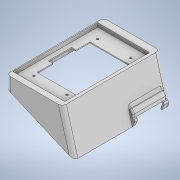
# Autodesk Inventor part: Front
Saved by Autodesk Inventor 2022 (Build 260153000, 153)
## iProperties
Created: 2021-06-27
Part Number: Front
Material: Generic
Document SubType Name: Modeling
Designer: Anton
Density: 1 g/cm^3
Appearance: Default
Author: Anton
Autodesk Inventor part; units mm, degrees
ref_plane "YZ Plane" through (0, 0, 0) normal (1, 0, 0) x (0, 1, 0)
ref_plane "XZ Plane" through (0, 0, 0) normal (0, 1, 0) x (-1, 0, 0)
ref_plane "XY Plane" through (0, 0, 0) normal (0, 0, 1) x (1, 0, 0)
sketch "Sketch1" plane through (0, 0, 0) normal (0, 1, 0) x (-1, 0, 0)
  line L0 (8, 0) -> (102.94, 0)
  line L1 (110.94, -8) -> (110.94, -185.2)
  line L2 (102.94, -193.2) -> (8, -193.2)
  line L3 (0, -185.2) -> (0, -8)
  circle A0 centre (88.297, -32) radius 2.1
  circle A1 centre (88.297, -158.2) radius 2.1
  circle A2 centre (22.6, -158.501) radius 2.1
  circle A3 centre (22.597, -32) radius 2.1
  arc A4 (110.94, -8) -> (102.94, 0) centre (102.94, -8) ccw
  arc A5 (8, 0) -> (0, -8) centre (8, -8) ccw
  arc A6 (0, -185.2) -> (8, -193.2) centre (8, -185.2) ccw
  arc A7 (102.94, -193.2) -> (110.94, -185.2) centre (102.94, -185.2) ccw
  point P0 (0, 0)
  dimension "d0" = 110.94
  dimension "d1" = 193.2
  dimension "d2" = 4.2
  dimension "d3" = 4.2
  dimension "d4" = 65.7
  dimension "d5" = 65.697
  dimension "d6" = 4.2
  dimension "d7" = 4.2
  dimension "d8" = 126.2
  dimension "d9" = 126.501
  dimension "d10" = 0
  dimension "d11" = 22.6
  dimension "d12" = 35
  dimension "d13" = 8
  dimension "d216" = 0
  dimension "d241" = 22.597
  constraints: 8 centre point, 8 end point, 8 point on circle, 8 tangent, 3 equal radius, 2 parallel, 2 point on line, 1 horizontal, 1 perpendicular
  measures "d0" distance between parallel lines of L3 L1
  measures "d1" distance between parallel lines of L2 L0
  measures "d2" diameter of A0
  measures "d3" diameter of A3
  measures "d4" distance of A3.centre A0.centre
  measures "d5" horizontal distance of A2.centre A1.centre
  measures "d6" diameter of A1
  measures "d7" diameter of A2
  measures "d8" distance of A1.centre A0.centre
  measures "d9" distance of A2.centre A3.centre
  measures "d10" vertical distance of A0.centre A3.centre
  measures "d11" distance from line of L3 A2.centre
  measures "d12" distance from line of L2 A1.centre
  measures "d13" radius of A4
  measures "d216" horizontal distance of A0.centre A1.centre
  measures "d241" distance from line of L3 A3.centre
extrude "Extrusion1" add sketch "Sketch1" along normal blind 2
sketch "Sketch2" plane through (0, 2, 0) normal (0, 1, 0) x (1, 0, 0)
  line L0 (-8, 193.2) -> (-102.94, 193.2) projected
  arc A0 (-102.94, 193.2) -> (-110.94, 185.2) centre (-102.94, 185.2) ccw projected
  line L1 (-110.94, 185.2) -> (-110.94, 8) projected
  arc A1 (-110.94, 8) -> (-102.94, 0) centre (-102.94, 8) ccw projected
  line L2 (-102.94, 0) -> (-8, 0) projected
  arc A2 (-8, 0) -> (0, 8) centre (-8, 8) ccw projected
  line L3 (0, 8) -> (0, 185.2) projected
  arc A3 (0, 185.2) -> (-8, 193.2) centre (-8, 185.2) ccw projected
  circle A4 centre (-88.297, 32) radius 2.1 projected
  circle A5 centre (-88.297, 158.2) radius 2.1 projected
  circle A6 centre (-22.6, 158.501) radius 2.1 projected
  circle A7 centre (-22.597, 32) radius 2.1 projected
  line L4 (-108.94, 11) -> (-108.94, 179.2)
  line L5 (-108.94, 179.2) -> (-6, 179.2)
  line L6 (-6, 11) -> (-108.94, 11)
  line L7 (-6, 179.2) -> (-6, 11)
  point P0 (0, 0)
  dimension "d16" = 2
  dimension "d17" = 14
  dimension "d18" = 11
  dimension "d19" = 6
  constraints: 8 end point, 1 horizontal
  measures "d16" distance between parallel lines of L1 L4
  measures "d17" distance between parallel lines of L0 L5
  measures "d18" distance between parallel lines of L2 L6
  measures "d19" distance between parallel lines of L3 L7
extrude "Extrusion2" add sketch "Sketch2" along normal blind 7.5 contours A3 L3 A2 L2 A1 L1 A0 L0
sketch "Sketch3" plane through (0, 2, 0) normal (0, 1, 0) x (1, 0, 0)
  line L0 (-91, 41) -> (-12, 41)
  line L1 (-12, 41) -> (-12, 146)
  line L2 (-12, 146) -> (-91, 146)
  line L3 (-6, 179.2) -> (-6, 11) projected
  line L4 (-6, 11) -> (-108.94, 11) projected
  line L5 (-99.94, 72) -> (-91, 72)
  line L6 (-91, 118.2) -> (-99.94, 118.2)
  line L7 (-99.94, 118.2) -> (-99.94, 72)
  circle A0 centre (-88.297, 158.2) radius 2.1 projected
  circle A1 centre (-88.297, 32) radius 2.1 projected
  line L8 (-108.94, 11) -> (-108.94, 179.2) projected
  line L9 (-91, 146) -> (-91, 118.2)
  line L10 (-91, 72) -> (-91, 41)
  point P0 (0, 0)
  dimension "d22" = 105
  dimension "d24" = 6
  dimension "d25" = 30
  dimension "d26" = 40
  dimension "d27" = 40
  dimension "d28" = 9
  constraints: 16 end point, 4 parallel, 2 horizontal, 1 perpendicular
  measures "d22" distance between parallel lines of L2 L0
  measures "d24" distance between parallel lines of L3 L1
  measures "d25" distance between parallel lines of L4 L0
  measures "d26" distance from line of L6 A0.centre
  measures "d27" distance from line of L5 A1.centre
  measures "d28" distance between parallel lines of L8 L7
extrude "Extrusion3" cut sketch "Sketch3" against normal blind 7.5 contours L10 L5 L7 L6 L9 L2 L1 L0
sketch "Sketch5" plane through (0, 0, 0) normal (0, -1, 0) x (1, 0, 0)
  line L0 (-12, -146) -> (-91, -146) projected
  line L1 (-91, -146) -> (-91, -118.2) projected
  line L2 (-91, -118.2) -> (-99.94, -118.2) projected
  line L3 (-99.94, -118.2) -> (-99.94, -72) projected
  line L4 (-99.94, -72) -> (-91, -72) projected
  line L5 (-91, -72) -> (-91, -41) projected
  line L6 (-91, -41) -> (-12, -41) projected
  line L7 (-12, -41) -> (-12, -146) projected
  line L8 (-8, -193.2) -> (-102.94, -193.2) projected
  arc A0 (-8, -193.2) -> (0, -185.2) centre (-8, -185.2) ccw projected
  line L9 (0, -8) -> (0, -185.2) projected
  arc A1 (0, -8) -> (-8, 0) centre (-8, -8) ccw projected
  line L10 (-102.94, 0) -> (-8, 0) projected
  arc A2 (-102.94, 0) -> (-110.94, -8) centre (-102.94, -8) ccw projected
  line L11 (-110.94, -185.2) -> (-110.94, -8) projected
  arc A3 (-110.94, -185.2) -> (-102.94, -193.2) centre (-102.94, -185.2) ccw projected
  circle A4 centre (-88.297, -32) radius 2.1 projected
  circle A5 centre (-88.297, -158.2) radius 2.1 projected
  circle A6 centre (-22.6, -158.501) radius 2.1 projected
  circle A7 centre (-22.597, -32) radius 2.1 projected
  line L12 (-102.94, -191.2) -> (-8, -191.2)
  arc A8 (-8, -191.2) -> (-2, -185.2) centre (-8, -185.2) ccw
  line L13 (-2, -185.2) -> (-2, -8)
  arc A9 (-2, -8) -> (-8, -2) centre (-8, -8) ccw
  line L14 (-8, -2) -> (-102.94, -2)
  arc A10 (-102.94, -2) -> (-108.94, -8) centre (-102.94, -8) ccw
  line L15 (-108.94, -8) -> (-108.94, -185.2)
  arc A11 (-108.94, -185.2) -> (-102.94, -191.2) centre (-102.94, -185.2) ccw
  point P0 (0, 0)
  dimension "d39" = 2
  constraints: 8 end point, 8 point on circle, 4 centre point, 7 other
  measures "d39" radial gap between concentric circles of A3 A11
extrude "Extrusion4" add sketch "Sketch5" along normal blind 72 contours L8 A3 L11 A2 L10 A1 L9 A0
sketch "Sketch6" plane through (-8, 9.5, -193.2) normal (0, 0, -1) x (-1, 0, 0)
  line L0 (102.94, -81.5) -> (102.94, 0)
  line L1 (-8, -81.5) -> (102.94, -81.5)
  line L2 (102.94, -81.5) -> (102.94, -23.5)
  line L3 (102.94, 0) -> (94.94, 0)
  line L4 (-8, -81.5) -> (0, -81.5)
  line L5 (0, 0) -> (-8, 0)
  line L6 (0, 0) -> (94.94, 0)
  line L7 (102.94, -23.5) -> (-25.549035, -79.092876)
  line L8 (-8, -81.5) -> (-29.89843, -81.5)
  line L9 (-29.89843, -81.5) -> (-31.1125, -81.5)
  line L10 (-25.549035, -79.092876) -> (-31.1125, -81.5)
  line L11 (-8, -81.5) -> (-8, 0)
  point P0 (-8, -9.5)
  dimension "d42" = 23.5
  dimension "d47" = 23.3965
  dimension "d48" = 140
  dimension "d51" = 23.1125
  constraints: 12 end point, 3 horizontal, 1 point on line
  measures "d42" distance from line of L3 L2.end
  measures "d47" angle of L6 L7
  measures "d48" distance of L2.end L7.end
  measures "d51" distance from line of L9.end L11
extrude "Extrusion5" cut sketch "Sketch6" along normal mid plane 1000 contours L1 L11 L7 L0 | L11 L8 L9 L10 L7
sketch "Sketch7" plane through (0, 9.5, 0) normal (0, 1, 0) x (1, 0, 0)
  arc A0 (-102.94, 193.2) -> (-110.94, 185.2) centre (-102.94, 185.2) ccw projected
  line L0 (-110.94, 185.2) -> (-110.94, 8) projected
  arc A1 (-110.94, 8) -> (-102.94, 0) centre (-102.94, 8) ccw projected
  line L1 (-102.94, 0) -> (-8, 0) projected
  arc A2 (-8, 0) -> (0, 8) centre (-8, 8) ccw projected
  line L2 (0, 8) -> (0, 185.2) projected
  arc A3 (0, 185.2) -> (-8, 193.2) centre (-8, 185.2) ccw projected
  line L3 (-8, 193.2) -> (-102.94, 193.2) projected
  line L4 (-108.94, 11) -> (-108.94, 179.2) projected
  line L5 (-108.94, 179.2) -> (-6, 179.2) projected
  line L6 (-6, 179.2) -> (-6, 11) projected
  line L7 (-6, 11) -> (-108.94, 11) projected
  line L8 (-8, 0) -> (23.113, 0)
  arc A4 (-8, 0) -> (0, 8) centre (-8, 8) ccw projected
  line L9 (23.113, 0) -> (23.113, 193.2)
  line L10 (23.113, 193.2) -> (-8, 193.2)
  arc A5 (0, 185.2) -> (-8, 193.2) centre (-8, 185.2) ccw projected
  point P0 (0, 0)
  point P1 (-8, 193.2)
  dimension "d52" = 23.113
  constraints: 6 end point, 2 perpendicular, 2 point on circle, 2 tangent, 1 horizontal
  measures "d52" distance between parallel lines of L2 L9
extrude "Extrusion6" add sketch "Sketch7" against normal up to surface contours L10 L9 L8 A2 L2 A3 surface through (-110.94, -14, -193.2) normal (0.397092, 0.9177788, 0)
sketch "Sketch8" plane through (-102.94, -17.46133, 0) normal (0, 0, 1) x (1, 0, 0)
  line L0 (126.053, 26.96133) -> (0, 26.96133)
  line L1 (126.053, 26.96133) -> (102.94, 26.96133)
  line L2 (0, 0) -> (126.053, -54.538886)
  line L3 (102.94, 26.96133) -> (126.053, -54.538886)
  line L4 (126.053, 26.96133) -> (126.053, -54.538886)
  line L5 (126.053, -54.538886) -> (126.053, 26.96133)
  point P0 (102.94, 17.46133)
  point P1 (96.94, 26.96133)
  dimension "d55" = 6
  constraints: 6 end point, 1 collinear, 1 point on line
  measures "d55" distance of point (96.94, 26.961) L1.end
extrude "Extrusion7" cut sketch "Sketch8" against normal blind 1000
sketch "Sketch9" plane through (0, 9.5, 0) normal (0, 1, 0) x (1, 0, 0)
  line L0 (23.113, 0) -> (0, 0) projected
  line L1 (-8, 0) -> (-110.94, 0)
  line L2 (-110.94, 0) -> (-110.94, 193.2)
  line L3 (-110.94, 193.2) -> (-8, 193.2)
  line L4 (0, 185.2) -> (0, 8)
  arc A0 (0, 185.2) -> (-8, 193.2) centre (-8, 185.2) ccw
  arc A1 (-8, 0) -> (0, 8) centre (-8, 8) ccw
  line L5 (0, 0) -> (0, 193.2) projected
  line L6 (0, 193.2) -> (0, 185.2)
  line L7 (-8, 193.2) -> (0, 193.2)
  line L8 (-102.94, 193.2) -> (23.113, 193.2) projected
  line L9 (-8, 0) -> (0, 0)
  line L10 (23.113, 0) -> (-102.94, 0) projected
  line L11 (0, 8) -> (0, 0)
  dimension "d58" = 8
  constraints: 16 end point, 6 tangent, 5 point on circle, 3 point on line, 2 centre point, 2 collinear, 2 parallel, 2 perpendicular, 1 equal radius, 1 horizontal
  measures "d58" radius of A0
sketch3d "3D Sketch1"
  line L0 (0, 9.5, 0) -> (23.113, -72.000216, 0)
sweep "Sweep1" cut profiles "Sketch9" path "3D Sketch1" contours A1 L5 L9 | A0 L7 L5
ref_plane "Work Plane1" through (23.113, -72.000216, -144.9) normal (-0.272835, 0.9620608, 0) x (0, 0, 1)
sketch "Sketch11" plane through (23.113, -72.000216, -144.9) normal (-0.272835, 0.9620608, 0) x (0, 0, 1)
  line L0 (-46.3, -106.390538) -> (-46.3, -26.259818)
  ellipse E0 centre (-40.3, -106.390538) end of major axis (-34.3, -106.390538) minor radius 5.064086 (-46.3, -106.390538) -> (-40.3, -111.454624) ccw
  line L1 (136.9, -111.454624) -> (-40.3, -111.454624)
  ellipse E1 centre (136.9, -106.390538) end of major axis (142.9, -106.390538) minor radius 5.064086 (136.9, -111.454624) -> (142.9, -106.390538) ccw
  line L2 (142.9, -26.259818) -> (142.9, -106.390538)
  ellipse E2 centre (136.9, -26.259818) end of major axis (130.9, -26.259818) minor radius 5.064086 (142.9, -26.259818) -> (136.9, -21.195732) ccw
  line L3 (-40.3, -21.195732) -> (136.9, -21.195732)
  ellipse E3 centre (-40.3, -26.259818) end of major axis (-46.3, -26.259818) minor radius 5.064086 (-40.3, -21.195732) -> (-46.3, -26.259818) ccw
  ellipse E4 centre (-40.3, -7.696487) end of major axis (-48.3, -7.696487) minor radius 7.696487 (-40.3, 0) -> (-48.3, -7.696487) ccw
  line L4 (-40.3, 0) -> (136.9, 0)
  ellipse E5 centre (136.9, -7.696487) end of major axis (144.9, -7.696487) minor radius 7.696487 (144.9, -7.696487) -> (136.9, 0) ccw
  line L5 (144.9, -7.696487) -> (144.9, -106.390538)
  ellipse E6 centre (136.9, -106.390538) end of major axis (144.9, -106.390538) minor radius 6.752115 (136.9, -113.142652) -> (144.9, -106.390538) ccw
  line L6 (-40.3, -113.142652) -> (136.9, -113.142652)
  ellipse E7 centre (-40.3, -106.390538) end of major axis (-32.3, -106.390538) minor radius 6.752115 (-48.3, -106.390538) -> (-40.3, -113.142652) ccw
  line L7 (-48.3, -106.390538) -> (-48.3, -7.696487)
  line L8 (142.9, -106.390538) -> (142.9, -7.696487)
  line L9 (136.9, -2) -> (-40.3, -2)
  line L10 (-46.3, -7.696487) -> (-46.3, -106.390538)
  line L11 (-40.3, -111.142652) -> (136.9, -111.142652)
  spline S0 degree 5 poles (142.900027, -7.696487) (142.900072, -6.800566) (142.71432, -5.904846) (142.342732, -5.060866) (141.262105, -3.534216) (139.68167, -2.526209) (138.783342, -2.175495) (137.841626, -2.000059) (136.9, -2.000018) knots 0 0 0 0 0 0 0.48753596 0.48753596 0.48753596 1 1 1 1 1 1
  spline S1 degree 5 poles (-40.3, -2.000018) (-41.241626, -2.000059) (-42.183342, -2.175495) (-43.08167, -2.526209) (-44.662105, -3.534216) (-45.742732, -5.060866) (-46.11432, -5.904846) (-46.300072, -6.800566) (-46.300027, -7.696487) knots 0 0 0 0 0 0 0.51246404 0.51246404 0.51246404 1 1 1 1 1 1
  spline S2 degree 5 poles (-46.300028, -106.390538) (-46.299997, -106.793405) (-46.245041, -107.196193) (-46.135378, -107.589075) (-45.689147, -108.646938) (-44.917064, -109.520861) (-44.327938, -109.984476) (-43.197488, -110.630825) (-41.951018, -110.989571) (-41.404874, -111.091631) (-40.852448, -111.14266) (-40.3, -111.142659) knots 0 0 0 0 0 0 0.23795953 0.23795953 0.23795953 0.67370232 0.67370232 0.67370232 1 1 1 1 1 1
  spline S3 degree 5 poles (136.9, -111.142659) (137.452448, -111.14266) (138.004874, -111.091631) (138.551018, -110.989571) (139.797488, -110.630825) (140.927938, -109.984476) (141.517064, -109.520861) (142.289147, -108.646938) (142.735378, -107.589075) (142.845041, -107.196193) (142.899997, -106.793405) (142.900028, -106.390538) knots 0 0 0 0 0 0 0.32629768 0.32629768 0.32629768 0.76204047 0.76204047 0.76204047 1 1 1 1 1 1
  point P0 (-46.3, -26.259818)
  dimension "d64" = 2
  constraints: 8 end point, 7 parallel, 20 other
  measures "d64" distance between parallel lines of L5 L8
extrude "Extrusion8" cut sketch "Sketch11" along normal up to surface contours L10 S1 L9 S0 L8 E2 L3 E3 surface through (-55.47, 0, -96.6) normal (0, 1, 0)
sketch "Sketch13" plane through (-110.94, -14, -185.2) normal (-0.397092, -0.9177788, 0) x (0.9177788, -0.397092, 0)
  line L0 (8.716697, -6) -> (136.126583, -6)
  ellipse E0 centre (8.716697, 0) end of major axis (15.25422, 0) minor radius 6 (2.179174, 0) -> (8.716697, -6) ccw
  line L1 (2.179174, 177.2) -> (2.179174, 0)
  ellipse E1 centre (8.716697, 177.2) end of major axis (15.25422, 177.2) minor radius 6 (8.716697, 183.2) -> (2.179174, 177.2) ccw
  line L2 (136.126583, 183.2) -> (8.716697, 183.2)
  spline S0 degree 7 poles (136.126583, 183.2) (136.514527, 183.200024) (136.902423, 183.180536) (137.289504, 183.141539) (137.674916, 183.082885) (138.05772, 183.004312) (138.436886, 182.905417) (139.157072, 182.674889) (139.498675, 182.546371) (139.835263, 182.39953) (140.165705, 182.233761) (140.488576, 182.048389) (140.802158, 181.842677) (141.299115, 181.469659) (141.489055, 181.314781) (141.673712, 181.15096) (141.852403, 180.977999) (142.024338, 180.795762) (142.188611, 180.604159) (142.457675, 180.256647) (142.566512, 180.105147) (142.670337, 179.948687) (142.768711, 179.787325) (142.861165, 179.621174) (142.947212, 179.450415) (143.149707, 179.002474) (143.25641, 178.71888) (143.344447, 178.425849) (143.412009, 178.125078) (143.457652, 177.818689) (143.480468, 177.509274) (143.480485, 177.2) knots 0 0 0 0 0 0 0 0 0.27563178 0.27563178 0.27563178 0.27563178 0.27563178 0.27563178 0.53020731 0.53020731 0.53020731 0.53020731 0.53020731 0.53020731 0.69417397 0.69417397 0.69417397 0.69417397 0.69417397 0.69417397 0.81372113 0.81372113 0.81372113 0.81372113 0.81372113 0.81372113 1 1 1 1 1 1 1 1
  line L3 (143.480508, 177.2) -> (143.480508, 0)
  spline S1 degree 7 poles (143.480508, 0) (143.480483, -0.309687) (143.457602, -0.619514) (143.411833, -0.926303) (143.344092, -1.227451) (143.255827, -1.520831) (143.148856, -1.804739) (142.945718, -2.253474) (142.859288, -2.424717) (142.766416, -2.591318) (142.667593, -2.753097) (142.563293, -2.90994) (142.453959, -3.06179) (142.184771, -3.408634) (142.020977, -3.599324) (141.849593, -3.780721) (141.671514, -3.952914) (141.487519, -4.116038) (141.298284, -4.270288) (140.803097, -4.641965) (140.49062, -4.847042) (140.168911, -5.031915) (139.839673, -5.197313) (139.504316, -5.343906) (139.163963, -5.472292) (138.443965, -5.703569) (138.063676, -5.80309) (137.679713, -5.882159) (137.293117, -5.941182) (136.904837, -5.980426) (136.515735, -6.000042) (136.126583, -6.000027) knots 0 0 0 0 0 0 0 0 0.18652709 0.18652709 0.18652709 0.18652709 0.18652709 0.18652709 0.30646281 0.30646281 0.30646281 0.30646281 0.30646281 0.30646281 0.46980351 0.46980351 0.46980351 0.46980351 0.46980351 0.46980351 0.72351021 0.72351021 0.72351021 0.72351021 0.72351021 0.72351021 1 1 1 1 1 1 1 1
  ellipse E2 centre (136.126583, 0) end of major axis (126.190741, 0) minor radius 8 (136.126583, -8) -> (146.062425, 0) ccw
  line L4 (146.062425, 0) -> (146.062425, 177.2)
  ellipse E3 centre (136.126583, 177.2) end of major axis (146.062425, 177.2) minor radius 8 (146.062425, 177.2) -> (136.126583, 185.2) ccw
  line L5 (136.126583, 185.2) -> (8.716697, 185.2)
  ellipse E4 centre (8.716697, 177.2) end of major axis (0, 177.2) minor radius 8 (8.716697, 185.2) -> (0, 177.2) ccw
  line L6 (0, 0) -> (0, 177.2)
  ellipse E5 centre (8.716697, 0) end of major axis (0, 0) minor radius 8 (0, 0) -> (8.716697, -8) ccw
  line L7 (8.716697, -8) -> (136.126583, -8)
  line L8 (91.389495, 183.2) -> (1.782943, 183.2)
  line L9 (15.179174, 175.2) -> (2.179174, 175.2)
  line L10 (2.179174, 177.2) -> (2.179174, 0)
  line L11 (15.179174, 183.2) -> (15.179174, 175.2)
  line L12 (-4.517914, 174.2) -> (89.958238, 174.2)
  line L13 (1.782943, -6) -> (91.389495, -6)
  line L14 (15.179174, -6) -> (15.179174, 2)
  line L15 (15.179174, 2) -> (2.179174, 2)
  line L16 (143.480508, 177.2) -> (143.480508, 0)
  line L17 (143.480508, 2) -> (126.480508, 2)
  line L18 (126.480508, 2) -> (126.480508, -6)
  line L19 (136.126583, -6) -> (91.389495, -6)
  line L20 (136.126583, 183.2) -> (91.389495, 183.2)
  line L21 (126.480508, 183.2) -> (126.480508, 175.2)
  line L22 (126.480508, 175.2) -> (143.480508, 175.2)
  point P0 (96.259095, 185.2)
  point P1 (143.480508, 2)
  point P2 (126.480508, -6)
  dimension "d80" = 13
  dimension "d81" = 8
  dimension "d82" = 8
  dimension "d83" = 13
  dimension "d84" = 17
  dimension "d85" = 8
  dimension "d86" = 8
  dimension "d87" = 17
  constraints: 16 end point, 8 point on line, 7 perpendicular, 8 other
  measures "d80" distance of L9.start L9.end
  measures "d81" distance of L11.start L9.start
  measures "d82" distance of L14.start L14.end
  measures "d83" distance of L14.end L15.end
  measures "d84" distance of L17.start L17.end
  measures "d85" distance of L17.end L18.end
  measures "d86" distance of L21.start L21.end
  measures "d87" distance of L21.end L22.end
sketch3d "3D Sketch2"
  line L0 (20.743372, -70.974958, -185.2) -> (0.615276, 0, -185.2)
sweep "Sweep2" add profiles "Sketch13" path "3D Sketch2" contours L18 L17 L3 S1 L0 | L22 L21 L2 S0 L3
sketch "Sketch14" plane through (-110.94, -14, -185.2) normal (-0.397092, -0.9177788, 0) x (0.9177788, -0.397092, 0)
  line L0 (8.716697, -6) -> (126.480508, -6)
  ellipse E0 centre (8.716697, 0) end of major axis (15.25422, 0) minor radius 6 (2.179174, 0) -> (8.716697, -6) ccw
  line L1 (2.179174, 177.2) -> (2.179174, 0)
  ellipse E1 centre (8.716697, 177.2) end of major axis (15.25422, 177.2) minor radius 6 (8.716697, 183.2) -> (2.179174, 177.2) ccw
  line L2 (126.480508, 183.2) -> (8.716697, 183.2)
  line L3 (126.480508, 183.2) -> (126.480508, 175.2)
  line L4 (126.480508, 175.2) -> (143.480508, 175.2)
  line L5 (143.480508, 175.2) -> (143.480508, 2)
  line L6 (143.480508, 2) -> (126.480508, 2)
  line L7 (126.480508, 2) -> (126.480508, -6)
  ellipse E2 centre (136.126583, 0) end of major axis (126.190741, 0) minor radius 8 (136.126583, -8) -> (146.062425, 0) ccw
  line L8 (146.062425, 0) -> (146.062425, 177.2)
  ellipse E3 centre (136.126583, 177.2) end of major axis (146.062425, 177.2) minor radius 8 (146.062425, 177.2) -> (136.126583, 185.2) ccw
  line L9 (136.126583, 185.2) -> (8.716697, 185.2)
  ellipse E4 centre (8.716697, 177.2) end of major axis (0, 177.2) minor radius 8 (8.716697, 185.2) -> (0, 177.2) ccw
  line L10 (0, 0) -> (0, 177.2)
  ellipse E5 centre (8.716697, 0) end of major axis (0, 0) minor radius 8 (0, 0) -> (8.716697, -8) ccw
  line L11 (8.716697, -8) -> (136.126583, -8)
  line L12 (8.716697, -6) -> (126.480508, -6)
  line L13 (15.179174, -6) -> (15.179174, 2)
  line L14 (15.179174, 2) -> (2.179174, 2)
  line L15 (84.261392, 183.2) -> (1.782943, 183.2)
  line L16 (15.179174, 183.2) -> (15.179174, 175.2)
  line L17 (15.179174, 175.2) -> (2.179174, 175.2)
  line L18 (2.179174, 177.2) -> (2.179174, 0)
  point P0 (96.259095, 185.2)
  point P1 (15.179174, -6)
  point P2 (15.179174, 183.2)
  dimension "d90" = 13
  dimension "d91" = 8
  dimension "d92" = 13
  dimension "d93" = 8
  constraints: 8 end point, 4 point on line, 2 perpendicular, 2 vertical, 6 other
  measures "d90" distance of L13.end L14.end
  measures "d91" distance of L13.start L13.end
  measures "d92" distance of L16.end L17.end
  measures "d93" distance of L16.start L16.end
extrude "Extrusion9" add sketch "Sketch14" against normal up to surface contours E0 L1 L14 L13 L0 | L1 E1 L2 L16 L17 surface through (-55.47, 0, -96.6) normal (0, 1, 0)
sketch "Sketch16" plane through (-110.94, -14, -185.2) normal (-0.397092, -0.9177788, 0) x (0.9177788, -0.397092, 0)
  ellipse E0 centre (8.716697, 0) end of major axis (15.25422, 0) minor radius 6 (2.179174, 0) -> (8.716697, -6) ccw
  line L0 (2.179174, 2) -> (2.179174, 0)
  line L1 (2.179174, 175.2) -> (2.179174, 2)
  line L2 (2.179174, 177.2) -> (2.179174, 175.2)
  ellipse E1 centre (8.716697, 177.2) end of major axis (15.25422, 177.2) minor radius 6 (8.716697, 183.2) -> (2.179174, 177.2) ccw
  line L3 (2.179174, 175.2) -> (15.179174, 175.2)
  line L4 (15.179174, 175.2) -> (15.179174, 183.2)
  line L5 (126.480508, 183.2) -> (15.179174, 183.2)
  line L6 (126.480508, 183.2) -> (126.480508, 175.2)
  line L7 (126.480508, 175.2) -> (143.480508, 175.2)
  line L8 (143.480508, 175.2) -> (143.480508, 2)
  line L9 (143.480508, 2) -> (126.480508, 2)
  line L10 (126.480508, 2) -> (126.480508, -6)
  line L11 (15.179174, -6) -> (126.480508, -6)
  line L12 (15.179174, -6) -> (15.179174, 2)
  line L13 (15.179174, 2) -> (2.179174, 2)
  ellipse E2 centre (136.126583, 0) end of major axis (126.190741, 0) minor radius 8 (136.126583, -8) -> (146.062425, 0) ccw
  line L14 (146.062425, 0) -> (146.062425, 177.2)
  ellipse E3 centre (136.126583, 177.2) end of major axis (146.062425, 177.2) minor radius 8 (146.062425, 177.2) -> (136.126583, 185.2) ccw
  line L15 (136.126583, 185.2) -> (8.716697, 185.2)
  ellipse E4 centre (8.716697, 177.2) end of major axis (0, 177.2) minor radius 8 (8.716697, 185.2) -> (0, 177.2) ccw
  line L16 (0, 0) -> (0, 177.2)
  ellipse E5 centre (8.716697, 0) end of major axis (0, 0) minor radius 8 (0, 0) -> (8.716697, -8) ccw
  line L17 (8.716697, -8) -> (136.126583, -8)
  line L18 (84.261392, 183.2) -> (15.179174, 183.2)
  line L19 (15.179174, 183.2) -> (10.681339, 185.2)
  line L20 (136.126583, 185.2) -> (8.716697, 185.2)
  line L21 (2.179174, 175.2) -> (2.179174, 2)
  line L22 (2.179174, 175.2) -> (0, 175.2)
  line L23 (2.179174, 2) -> (0, 2)
  line L24 (0, 0) -> (0, 177.2)
  line L25 (15.179174, -6) -> (15.179174, -8)
  point P0 (96.259095, 185.2)
  point P1 (0, 2)
  point P2 (10.681339, 185.2)
  constraints: 8 end point, 4 point on line, 2 perpendicular, 1 horizontal, 6 other
sketch3d "3D Sketch4"
  line L0 (-102.94, -17.46133, -193.2) -> (-102.94, 9.5, -193.2)
sweep "Sweep4" add profiles "Sketch16" path "3D Sketch4" contours L22 L16 E4 L15 L19 L4 L3 | L13 L12 L25 L17 E5 L16 L23
sketch "Sketch17" plane through (-102.94, 9.5, 0) normal (0, 0, 1) x (1, 0, 0)
  line L0 (-6, 0) -> (96.94, 0)
  line L1 (0.651334, 0) -> (-10.950473, 0)
  line L2 (-10.950473, 0) -> (-10.950473, 5.742585)
  line L3 (-10.950473, 5.742585) -> (0.651334, 5.742585)
  line L4 (0.651334, 5.742585) -> (0.651334, 0)
  point P0 (102.94, -9.5)
  constraints: 8 end point, 2 parallel, 1 horizontal, 1 perpendicular, 1 point on line
extrude "Extrusion10" cut sketch "Sketch17" along normal mid plane 1000
sketch "Sketch18" plane through (-110.94, -14, -185.2) normal (-0.397092, -0.9177788, 0) x (0.9177788, -0.397092, 0)
  circle A0 centre (10, -2.5) radius 2.1
  circle A1 centre (10, 179.7) radius 2.1
  circle A2 centre (133.062425, 179.7) radius 2.1
  circle A3 centre (133.062425, -2.5) radius 2.1
  line L0 (8.716697, -8) -> (136.126583, -8)
  line L1 (146.062425, 0) -> (146.062425, 177.2)
  line L2 (0, 0) -> (0, 177.2)
  line L3 (136.126583, 185.2) -> (8.716697, 185.2)
  point P0 (96.259095, 185.2)
  dimension "d26" = 40
  dimension "d102" = 4.2
  dimension "d103" = 5.5
  dimension "d104" = 13
  dimension "d105" = 4.2
  dimension "d106" = 4.2
  dimension "d107" = 4.2
  dimension "d108" = 10
  dimension "d109" = 5.5
  dimension "d110" = 5.5
  dimension "d111" = 10
  dimension "d112" = 13
  dimension "d113" = 5.5
  constraints: 4 centre point
  measures "d102" diameter of A3
  measures "d103" distance from line of L0 A3.centre
  measures "d104" distance from line of L1 A3.centre
  measures "d105" diameter of A2
  measures "d106" diameter of A1
  measures "d107" diameter of A0
  measures "d108" distance from line of L2 A0.centre
  measures "d109" distance from line of L0 A0.centre
  measures "d110" distance from line of L3 A1.centre
  measures "d111" distance from line of L2 A1.centre
  measures "d112" distance from line of L1 A2.centre
  measures "d113" distance from line of L3 A2.centre
extrude "Extrusion11" cut sketch "Sketch18" against normal blind 9
chamfer "Chamfer1" distance 0.8 angle 45 4 edges at (9.2545, -66.0041, -187.7) (-103.6895, -17.137, -187.7) (9.2545, -66.0041, -5.5) (-103.6895, -17.137, -5.5)
sketch "Sketch23" plane through (-13.072543, 0, -183.2) normal (0, 0, 1) x (1, 0, 0)
  line L0 (33.815915, -70.974958) -> (18.213675, -64.224395)
  line L1 (0, 0) -> (13.687818, 0)
  line L2 (18.213675, -64.224395) -> (13.687818, 0)
  line L3 (13.687818, 0) -> (0, 0)
  line L4 (18.213675, -64.224395) -> (0, 0)
  line L5 (0, 0) -> (18.213675, -64.224395)
  point P0 (13.072543, 0)
  constraints: 6 end point, 2 collinear
extrude "Extrusion12" cut sketch "Sketch23" against normal up to surface (8 mm away)
sketch "Sketch24" plane through (0.615276, 0, -10) normal (0, 0, -1) x (-1, 0, 0)
  line L0 (0, 0) -> (13.687818, 0)
  line L1 (-4.525856, -64.224395) -> (0, 0)
  line L2 (0, 0) -> (13.687818, 0)
  line L3 (-4.525856, -64.224395) -> (-20.128096, -70.974958)
  line L4 (13.687818, 0) -> (-4.525856, -64.224395)
  point P0 (0.615276, 0)
  constraints: 6 end point, 1 collinear
extrude "Extrusion13" cut sketch "Sketch24" against normal up to surface (8 mm away)
sketch "Sketch28" plane through (0, 9.5, 0) normal (0, 1, 0) x (1, 0, 0)
  line L0 (-108.94, 179.2) -> (-6, 179.2)
  line L1 (-6, 179.2) -> (-6, 11)
  line L2 (-6, 11) -> (-108.94, 11)
  line L3 (-108.94, 11) -> (-108.94, 179.2)
  line L4 (-8, 193.2) -> (-102.94, 193.2)
  arc A0 (-102.94, 193.2) -> (-110.94, 185.2) centre (-102.94, 185.2) ccw
  line L5 (-110.94, 185.2) -> (-110.94, 8)
  arc A1 (-110.94, 8) -> (-102.94, 0) centre (-102.94, 8) ccw
  line L6 (-102.94, 0) -> (-8, 0)
  arc A2 (-8, 0) -> (0, 8) centre (-8, 8) ccw
  line L7 (0, 8) -> (0, 185.2)
  arc A3 (0, 185.2) -> (-8, 193.2) centre (-8, 185.2) ccw
  line L8 (-8, 191.2) -> (-102.94, 191.2)
  arc A4 (-102.94, 191.2) -> (-108.94, 185.2) centre (-102.94, 185.2) ccw
  line L9 (-108.94, 185.2) -> (-108.94, 8)
  arc A5 (-108.94, 8) -> (-102.94, 2) centre (-102.94, 8) ccw
  line L10 (-102.94, 2) -> (-8, 2)
  arc A6 (-8, 2) -> (-2, 8) centre (-8, 8) ccw
  line L11 (-2, 8) -> (-2, 185.2)
  arc A7 (-2, 185.2) -> (-8, 191.2) centre (-8, 185.2) ccw
  line L12 (-10.533536, 193.2) -> (-10.533536, 191.2)
  line L13 (-88.343639, 191.2) -> (-0.014351, 191.2)
  line L14 (-0.014351, 2) -> (-88.343639, 2)
  line L15 (-15.654738, 2) -> (-15.654738, 0)
  point P0 (0, 0)
  dimension "d127" = 2
  constraints: 12 end point, 8 point on circle, 4 centre point, 4 point on line, 2 perpendicular, 7 other
  measures "d127" radial gap between concentric circles of A3 A7
sketch3d "3D Sketch5"
  line L0 (0, 9.5, -8) -> (23.113, -72.000216, -8)
sweep "Sweep5" add profiles "Sketch28" path "3D Sketch5" contours L12 L4 A3 L13 L8 | L10 L14 A2 L6 L15 | L13 A3 L7 A2 L14 A6 L11 A7
sketch "Sketch29" plane through (-102.94, -17.46133, 0) normal (0, 0, 1) x (1, 0, 0)
  line L0 (108.081132, -46.763064) -> (5.931125, -2.566198)
  line L1 (104.775828, -45.33297) -> (127.217667, -55.042798)
  line L2 (127.217667, -55.042798) -> (105.606273, -56.239092)
  line L3 (105.606273, -56.239092) -> (104.775828, -45.33297)
  point P0 (102.94, 17.46133)
  point P1 (108.081132, -46.763064)
  constraints: 6 end point, 1 collinear, 1 point on line
extrude "Extrusion14" cut sketch "Sketch29" along normal mid plane 1000
sketch "Sketch31" plane through (-110.94, -14, -185.2) normal (-0.397092, -0.9177788, 0) x (0.9177788, -0.397092, 0)
  line L0 (146.062425, 2) -> (74.476425, 2)
  line L1 (74.476425, 2) -> (74.476425, 69.15)
  line L2 (74.476425, 69.15) -> (146.062425, 69.15)
  line L3 (146.062425, 69.15) -> (146.062425, 2)
  line L4 (146.062425, 0) -> (146.062425, 177.2)
  line L5 (143.480508, 2) -> (126.480508, 2)
  point P0 (96.259095, 185.2)
  dimension "d133" = 71.586
  dimension "d134" = 67.15
  dimension "d135" = 0
  dimension "d136" = 0
  constraints: 8 end point, 2 parallel, 1 horizontal, 1 perpendicular
  measures "d133" distance between parallel lines of L1 L3
  measures "d134" distance between parallel lines of L2 L0
  measures "d135" distance between parallel lines of L4 L3
  measures "d136" distance between parallel lines of L5 L0
extrude "Extrusion15" cut sketch "Sketch31" against normal blind 16
sketch "Sketch46" plane through (23.113, -72.000216, -116.05) normal (0, 0, -1) x (-0.9177788, 0.397092, 0)
  line L0 (0, 0) -> (3, 0)
  line L1 (9.935842, 0) -> (0, 0)
  line L2 (3, 0) -> (3, 12.17)
  line L3 (0, 0) -> (0, 14.17)
  line L4 (0, 14.17) -> (3, 14.17)
  line L5 (0, 14.17) -> (5, 14.17)
  line L6 (5, 14.17) -> (7.538743, 19.572444)
  line L7 (20.682372, 22.17) -> (11.248336, 22.17)
  line L8 (3, 12.17) -> (6.2, 12.17)
  line L9 (6.2, 12.17) -> (9.239811, 18.638717)
  line L10 (9.248367, 20.181094) -> (9.239811, 18.638717)
  arc A0 (11.248336, 22.17) -> (9.248367, 20.181094) centre (11.248336, 20.17) ccw
  line L11 (0, 0) -> (53.575704, 65.621186)
  line L12 (22.13413, 27.110569) -> (28.356172, 34.73152)
  line L13 (2.581916, 0) -> (49.238643, 57.146608)
  line L14 (29.905409, 33.466662) -> (22.31525, 24.17)
  line L15 (14.779142, 24.17) -> (15.937182, 24.17)
  line L16 (22.31525, 24.17) -> (20.682372, 22.17)
  arc A1 (15.937182, 24.17) -> (22.13413, 27.110569) centre (15.937182, 32.17) ccw
  arc A2 (14.779142, 24.17) -> (7.538743, 19.572444) centre (14.779142, 16.17) ccw
  point P0 (49.80333, 56.902287)
  point P1 (9.699249, 24.17)
  point P2 (19.733334, 24.17)
  point P3 (3, 3.674493)
  point P4 (18.100455, 22.17)
  point P5 (22.13413, 27.110569)
  point P6 (3, 14.17)
  dimension "d175" = 14.17
  dimension "d176" = 3
  dimension "d178" = 5
  dimension "d179" = 115.17
  dimension "d180" = 10
  dimension "d183" = 2
  dimension "d184" = 115.17
  dimension "d185" = 3.2
  dimension "d187" = 2
  dimension "d188" = 8
  constraints: 28 end point, 10 point on line, 6 point on circle, 5 tangent, 4 horizontal, 3 centre point, 2 perpendicular, 1 equal radius, 1 vertical
  measures "d175" distance of L0.end L4.end
  measures "d176" distance between parallel lines of L3 L2
  measures "d178" distance of L3.end L5.end
  measures "d179" angle of L5 L6
  measures "d180" vertical distance of L5.end point (9.699, 24.17)
  measures "d183" distance between parallel lines of L8 L5
  measures "d184" angle of L8 L9
  measures "d185" distance of L2.end L8.end
  measures "d187" radius of A0
  measures "d188" radius of A1
extrude "Extrusion24" add sketch "Sketch46" along normal up to surface (67.15 mm away) contours L3 L4 L5 L6 A2 L15 A1 L11 L7 A0 L10 L9 L8 L2
sketch "Sketch47" plane through (23.113, -72.000216, -183.2) normal (0, 0, -1) x (-0.9177788, 0.397092, 0)
  line L0 (0, 14.17) -> (0, 0)
  line L1 (3, 3.674493) -> (0, 0)
  line L2 (3, 3.674493) -> (3, 12.17)
  line L3 (3, 12.17) -> (6.2, 12.17)
  line L4 (6.2, 12.17) -> (9.239811, 18.638717)
  line L5 (9.239811, 18.638717) -> (9.248367, 20.181094)
  arc A0 (11.248336, 22.17) -> (9.248367, 20.181094) centre (11.248336, 20.17) ccw
  line L6 (11.248336, 22.17) -> (18.100455, 22.17)
  line L7 (22.13413, 27.110569) -> (18.100455, 22.17)
  arc A1 (15.937182, 24.17) -> (22.13413, 27.110569) centre (15.937182, 32.17) ccw
  line L8 (15.937182, 24.17) -> (14.779142, 24.17)
  arc A2 (14.779142, 24.17) -> (7.538743, 19.572444) centre (14.779142, 16.17) ccw
  line L9 (7.538743, 19.572444) -> (5, 14.17)
  line L10 (5, 14.17) -> (0, 14.17)
  line L11 (11.248336, 22.17) -> (18.100455, 22.17)
  line L12 (3, 3.674493) -> (13.063026, 16)
  line L13 (3, 3.674493) -> (18.100455, 22.17)
  point P0 (49.80333, 56.902287)
  point P1 (13.063026, 16)
  point P2 (18.100455, 22.17)
  constraints: 2 end point, 2 point on line
extrude "Extrusion25" add sketch "Sketch47" against normal blind 2 contours L2 L3 L4 L5 A0 L6 L13 L12
sketch "Sketch48" plane through (23.113, -72.000216, -116.05) normal (0, 0, 1) x (0.9177788, -0.397092, 0)
  line L0 (-15.937182, 24.17) -> (-14.779142, 24.17)
  line L1 (0, 0) -> (-3, 3.674493)
  line L2 (0, 14.17) -> (0, 0)
  line L3 (-5, 14.17) -> (0, 14.17)
  line L4 (-7.538743, 19.572444) -> (-5, 14.17)
  arc A0 (-7.538743, 19.572444) -> (-14.779142, 24.17) centre (-14.779142, 16.17) ccw
  line L5 (-15.937182, 24.17) -> (-14.779142, 24.17)
  arc A1 (-22.13413, 27.110569) -> (-15.937182, 24.17) centre (-15.937182, 32.17) ccw
  line L6 (-18.100455, 22.17) -> (-22.13413, 27.110569)
  line L7 (-11.248336, 22.17) -> (-18.100455, 22.17)
  arc A2 (-9.248367, 20.181094) -> (-11.248336, 22.17) centre (-11.248336, 20.17) ccw
  line L8 (-9.239811, 18.638717) -> (-9.248367, 20.181094)
  line L9 (-6.2, 12.17) -> (-9.239811, 18.638717)
  line L10 (-3, 12.17) -> (-6.2, 12.17)
  line L11 (-3, 3.674493) -> (-3, 12.17)
  line L12 (-13.063026, 16) -> (-3, 3.674493)
  line L13 (-3, 3.674493) -> (-18.100455, 22.17)
  point P0 (-49.80333, 56.902287)
  point P1 (-13.063026, 16)
  constraints: 2 end point, 1 collinear
extrude "Extrusion26" add sketch "Sketch48" against normal blind 2 contours L7 A2 L8 L9 L10 L11 L12 L13
fillet "Fillet1" radius 3 8 edges at (24.0585, -54.0266, -183.2) (18.6153, -43.7189, -183.2) (15.243, -41.4182, -183.2) (22.5875, -46.7957, -183.2) (24.0585, -54.0266, -116.05) (18.6153, -43.7189, -116.05) (15.243, -41.4182, -116.05) (22.5875, -46.7957, -116.05)
sketch "Sketch50" plane through (23.113, -72.000216, -181.2) normal (0, 0, 1) x (0.9177788, -0.397092, 0)
  line L0 (0, 0) -> (-53.575704, 65.621186)
  line L1 (-12.566014, 15.391244) -> (-21.259598, 15.391244)
  line L2 (-21.259598, 15.391244) -> (-21.259598, 22.17)
  line L3 (-21.259598, 22.17) -> (-12.566014, 22.17)
  line L4 (-12.566014, 22.17) -> (-12.566014, 15.391244)
  point P0 (-49.80333, 56.902287)
  constraints: 8 end point, 2 parallel, 1 horizontal, 1 perpendicular, 1 point on line
extrude "Extrusion27" cut sketch "Sketch50" along normal up to surface (63.15 mm away)
sketch "Sketch51" plane through (28.739793, -58.99529, -116.05) normal (0.9177788, -0.397092, 0) x (0, 0, -1)
  line L0 (3, 0) -> (64.15, 0) projected
  line L1 (0, -14.17) -> (67.15, -14.17) projected
  line L2 (58.15, 0) -> (5.65, 0)
  line L3 (5.65, 0) -> (5.65, -14.17)
  line L4 (5.65, -14.17) -> (58.15, -14.17)
  line L5 (58.15, -14.17) -> (58.15, 0)
  line L6 (67.15, 0) -> (67.15, -14.17) projected
  line L7 (0, 0) -> (0, -14.17) projected
  point P0 (-116.05, 42.732287)
  point P1 (58.15, -14.17)
  point P2 (5.65, 0)
  dimension "d198" = 9
  dimension "d199" = 5.65
  constraints: 8 end point, 2 parallel, 2 point on line, 1 horizontal, 1 perpendicular
  measures "d198" distance between parallel lines of L6 L5
  measures "d199" distance between parallel lines of L7 L3
extrude "Extrusion28" cut sketch "Sketch51" against normal blind 10
fillet "Fillet2" radius 3 2 edges at (28.7398, -58.9953, -118.875) (28.7398, -58.9953, -178.7)
sketch "Sketch52" plane through (-88.343639, 0, -191.2) normal (0, 0, 1) x (1, 0, 0)
  line L0 (-8.665237, -20.027528) -> (93.484771, -64.224395)
  line L1 (14.279234, -29.954828) -> (17.654516, -22.153708)
  line L2 (17.654516, -22.153708) -> (2.970054, -15.800236)
  line L3 (2.970054, -15.800236) -> (-0.405227, -23.601356)
  line L4 (0, 0) -> (-8.665237, -20.027528)
  point P0 (88.343639, 0)
  dimension "d203" = 9
  dimension "d204" = 8.5
  dimension "d209" = 16
  constraints: 6 end point, 2 perpendicular, 2 point on line
  measures "d203" distance between parallel lines of L4 L3
  measures "d204" distance between parallel lines of L2 L0
  measures "d209" distance between parallel lines of L3 L1
extrude "Extrusion29" cut sketch "Sketch52" against normal blind 1.5
sketch "Sketch53" plane through (-88.343639, 0, -192.7) normal (0, 0, 1) x (1, 0, 0)
  line L0 (13.562632, -28.337273) -> (15.865765, -23.014156)
  line L1 (17.654516, -22.153708) -> (14.279234, -29.954828)
  line L2 (15.865765, -23.014156) -> (3.567529, -17.693124)
  line L3 (3.567529, -17.693124) -> (1.264396, -23.016241)
  line L4 (1.264396, -23.016241) -> (13.562632, -28.337273)
  line L5 (2.970054, -15.800236) -> (17.654516, -22.153708)
  line L6 (-0.405227, -23.601356) -> (2.970054, -15.800236)
  point P0 (88.343639, 0)
  dimension "d207" = 5.8
  dimension "d208" = 13.4
  dimension "d210" = 1.5
  dimension "d211" = 1.3
  constraints: 8 end point, 2 perpendicular, 1 parallel
  measures "d207" distance between parallel lines of L2 L4
  measures "d208" distance between parallel lines of L3 L0
  measures "d210" distance between parallel lines of L5 L2
  measures "d211" distance between parallel lines of L6 L3
extrude "Extrusion30" cut sketch "Sketch53" against normal blind 1.5
sketch "Sketch57" plane through (-88.343639, 0, -191.2) normal (0, 0, 1) x (1, 0, 0)
  line L0 (-14.596361, -17.46133) -> (102.337733, -68.054773)
  line L1 (31.60396, -33.855015) -> (26.647954, -31.710719)
  line L2 (26.127268, -30.395848) -> (26.643487, -29.202735)
  line L3 (26.643487, -29.202735) -> (33.43505, -32.141216)
  line L4 (33.43505, -32.141216) -> (32.918831, -33.334328)
  line L5 (31.60396, -33.855015) -> (32.918831, -33.334328)
  line L6 (26.647954, -31.710719) -> (26.127268, -30.395848)
  line L7 (17.654516, -22.153708) -> (14.279234, -29.954828)
  line L8 (-0.405227, -23.601356) -> (2.970054, -15.800236)
  line L9 (14.279234, -29.954828) -> (-0.405227, -23.601356)
  line L10 (6.937003, -26.778092) -> (9.142085, -21.681597)
  line L11 (3.567529, -17.693124) -> (15.865765, -23.014156)
  point P0 (88.343639, 0)
  dimension "d217" = 7.4
  dimension "d218" = 2.3
  dimension "d222" = 135
  dimension "d223" = 135
  dimension "d224" = 1.31487
  dimension "d225" = 1.31487
  dimension "d226" = 8
  dimension "d227" = 19.049
  dimension "d228" = 3.3
  constraints: 16 end point, 5 perpendicular, 1 midpoint
  measures "d217" distance between parallel lines of L2 L4
  measures "d218" distance between parallel lines of L3 L1
  measures "d222" angle of L1 L5
  measures "d223" angle of L1 L6
  measures "d224" horizontal distance of L1.start L4.end
  measures "d225" vertical distance of L1.end L2.start
  measures "d226" distance between parallel lines of L10 L8
  measures "d227" distance between parallel lines of L2 L10
  measures "d228" distance between parallel lines of L0 L1
extrude "Extrusion31" cut sketch "Sketch57" against normal blind 10
sketch "Sketch58" plane through (-88.343639, 0, -191.2) normal (0, 0, 1) x (1, 0, 0)
  line L0 (14.279234, -29.954828) -> (93.484771, -64.224395)
  line L1 (35.066006, -38.948564) -> (36.495537, -35.64456)
  line L2 (36.495537, -35.64456) -> (21.994632, -29.370507)
  line L3 (21.994632, -29.370507) -> (20.565101, -32.67451)
  line L4 (33.43505, -32.141216) -> (32.918831, -33.334328)
  line L5 (26.127268, -30.395848) -> (26.643487, -29.202735)
  line L6 (33.558645, -34.373866) -> (34.749921, -31.620529)
  line L7 (34.749921, -31.620529) -> (26.1228, -27.887865)
  line L8 (26.1228, -27.887865) -> (24.931524, -30.641201)
  line L9 (26.643487, -29.202735) -> (33.43505, -32.141216)
  point P0 (88.343639, 0)
  dimension "d231" = 15.8
  dimension "d232" = 4.2
  dimension "d233" = 4.2
  dimension "d234" = 3.6
  dimension "d235" = 1
  dimension "d236" = 1
  dimension "d237" = 1
  constraints: 12 end point, 6 perpendicular, 4 point on line
  measures "d231" distance between parallel lines of L3 L1
  measures "d232" distance between parallel lines of L4 L1
  measures "d233" distance between parallel lines of L5 L3
  measures "d234" distance between parallel lines of L0 L2
  measures "d235" distance between parallel lines of L4 L6
  measures "d236" distance between parallel lines of L5 L8
  measures "d237" distance between parallel lines of L9 L7
extrude "Extrusion32" cut sketch "Sketch58" against normal blind 1.5
sketch "Sketch60" plane through (0.615276, 0, -183.2) normal (-0.9620608, -0.272835, 0) x (0, 0, 1)
  line L0 (67.15, -75.406755) -> (175.2, -75.406755)
  line L1 (65.15, -53.118547) -> (67.15, -53.118547)
  line L2 (67.15, -75.406755) -> (65.15, -75.406755)
  line L3 (65.15, -75.406755) -> (65.15, -53.118547)
  line L4 (65.15, -53.118547) -> (67.15, -53.118547)
  line L5 (67.15, -53.118547) -> (67.15, -75.406755)
  line L6 (0, -54.751426) -> (0, -75.406755)
  line L7 (0, -53.118547) -> (2, -53.118547)
  line L8 (0, -75.406755) -> (2, -75.406755)
  line L9 (2, -75.406755) -> (2, -53.118547)
  line L10 (2, -53.118547) -> (0, -53.118547)
  line L11 (0, -53.118547) -> (0, -75.406755)
  point P0 (183.2, 0.167869)
  point P1 (0, -53.118547)
  constraints: 16 end point, 4 parallel, 2 horizontal, 2 perpendicular
extrude "Extrusion33" add sketch "Sketch60" against normal up to surface (2 mm away)
sketch "Sketch61" plane through (20.743372, -70.974958, -10) normal (0, 0, -1) x (-0.9177788, 0.397092, 0)
  line L0 (17, 0) -> (0, 0)
  line L1 (1.662219, 0) -> (-3.33995, 0)
  line L2 (-3.33995, 0) -> (-3.33995, -2.986506)
  line L3 (-3.33995, -2.986506) -> (1.662219, -2.986506)
  line L4 (1.662219, -2.986506) -> (1.662219, 0)
  point P0 (47.221414, 56.902287)
  constraints: 8 end point, 2 parallel, 1 horizontal, 1 perpendicular, 1 point on line
extrude "Extrusion34" cut sketch "Sketch61" along normal mid plane 1000
sketch "Sketch62" plane through (-110.94, -14, -185.2) normal (-0.397092, -0.9177788, 0) x (0.9177788, -0.397092, 0)
  line L0 (146.062425, 67.15) -> (146.062425, 63.5)
  line L1 (143.480508, 175.2) -> (143.480508, 67.15)
  line L2 (146.062425, 63.5) -> (143.480508, 63.5)
  line L3 (143.480508, 63.5) -> (143.480508, 67.15)
  line L4 (143.480508, 67.15) -> (146.062425, 67.15)
  line L5 (146.062425, 67.15) -> (146.062425, 63.5)
  line L6 (146.062425, 11) -> (143.062425, 11)
  line L7 (143.062425, 4) -> (146.062425, 4)
  line L8 (146.062425, 11) -> (143.480508, 11)
  line L9 (143.480508, 11) -> (143.480508, 4)
  line L10 (143.480508, 4) -> (146.062425, 4)
  line L11 (146.062425, 4) -> (146.062425, 11)
  point P0 (96.259095, 185.2)
  point P1 (146.062425, 67.15)
  point P2 (146.062425, 4)
  point P3 (143.480508, 11)
  constraints: 16 end point, 4 parallel, 2 horizontal, 2 perpendicular, 2 point on line
extrude "Extrusion35" add sketch "Sketch62" against normal blind 10
body "Solid1"
